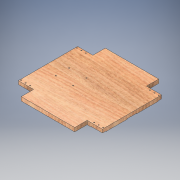
# Autodesk Inventor part: BottomPlateV1
Saved by Autodesk Inventor 2017 (Build 210142000, 142)
## iProperties
Created: 2017-01-25
Part Number: BottomPlateV1
Material: Wood (Birch)
Document SubType Name: Modeling
Designer: Naga
Density: 0.55 g/cm^3
Appearance: Birch - Natural Polished
Author: Naga
Autodesk Inventor part; units mm, degrees
ref_plane "YZ Plane" through (0, 0, 0) normal (1, 0, 0) x (0, 1, 0)
ref_plane "XZ Plane" through (0, 0, 0) normal (0, 1, 0) x (-1, 0, 0)
ref_plane "XY Plane" through (0, 0, 0) normal (0, 0, 1) x (1, 0, 0)
sketch "Sketch1" plane through (0, 0, 0) normal (0, 1, 0) x (-1, 0, 0)
  line L0 (-279.4, -127.4986) -> (-279.4, -151.8986)
  line L1 (-277.4, -125.4986) -> (-174.3, -125.4986)
  line L2 (-174.3, -153.8986) -> (-277.4, -153.8986)
  circle A0 centre (-275.8, -47.0543) radius 1.25
  circle A1 centre (-261, -47.0543) radius 1.25
  circle A2 centre (-246.2, -47.0543) radius 1.25
  circle A3 centre (-261, -232.44) radius 1.25
  circle A4 centre (-18.4, -47.0543) radius 1.25
  circle A5 centre (-48.23, -117.9957) radius 1.778
  circle A6 centre (-48.23, -162.1917) radius 1.778
  circle A7 centre (-105.38, -162.1917) radius 1.778
  circle A8 centre (-105.38, -117.9957) radius 1.778
  line L3 (0, 0) -> (-279.4, 0)
  line L4 (-279.4, 0) -> (-279.4, -279.4)
  line L5 (-279.4, -279.4) -> (0, -279.4)
  line L6 (0, -279.4) -> (0, 0)
  line L7 (-279.4, 0) -> (-228.6, 0)
  line L8 (-228.6, 0) -> (-228.6, -41.275)
  line L9 (-228.6, -41.275) -> (-279.4, -41.275)
  line L10 (-279.4, -41.275) -> (-279.4, 0)
  line L11 (-279.4, -279.4) -> (-228.6, -279.4)
  line L12 (-228.6, -279.4) -> (-228.6, -238.125)
  line L13 (-228.6, -238.125) -> (-279.4, -238.125)
  line L14 (-279.4, -238.125) -> (-279.4, -279.4)
  line L15 (0, -279.4) -> (-50.8, -279.4)
  line L16 (-50.8, -279.4) -> (-50.8, -238.125)
  line L17 (-50.8, -238.125) -> (0, -238.125)
  line L18 (0, -238.125) -> (0, -279.4)
  line L19 (0, 0) -> (-50.8, 0)
  line L20 (-50.8, 0) -> (-50.8, -41.275)
  line L21 (-50.8, -41.275) -> (0, -41.275)
  line L22 (0, -41.275) -> (0, 0)
  arc A9 (-174.3, -153.6986) -> (-174.3, -125.6986) centre (-182.3, -139.6986) ccw
  line L23 (-162.35, -123.8236) -> (-289.35, -123.8236)
  line L24 (-289.35, -123.8236) -> (-289.35, -155.5736)
  line L25 (-289.35, -155.5736) -> (-162.35, -155.5736)
  line L26 (-162.35, -155.5736) -> (-162.35, -123.8236)
  line L27 (-162.35, -123.8236) -> (-289.35, -155.5736) construction
  line L28 (-289.35, -123.8236) -> (-162.35, -155.5736) construction
  line L29 (-280.05, -238.79) -> (-241.95, -238.79)
  line L30 (-241.95, -238.79) -> (-241.95, -226.09)
  line L31 (-241.95, -226.09) -> (-280.05, -226.09)
  line L32 (-280.05, -226.09) -> (-280.05, -238.79)
  line L33 (-280.05, -238.79) -> (-241.95, -226.09) construction
  line L34 (-241.95, -238.79) -> (-280.05, -226.09) construction
  circle A10 centre (-261, -232.44) radius 1.5875
  circle A11 centre (-246.2, -232.44) radius 1.5875
  circle A12 centre (-275.8, -232.44) radius 1.5875
  line L35 (-261, -47.0543) -> (-261, -232.44)
  line L36 (-261, -232.44) -> (-18.4, -232.44)
  circle A13 centre (-261, -47.0454) radius 1.5875
  line L37 (-280.05, -53.3954) -> (-241.95, -53.3954)
  line L38 (-241.95, -53.3954) -> (-241.95, -40.6954)
  line L39 (-241.95, -40.6954) -> (-280.05, -40.6954)
  circle A14 centre (-246.2, -47.0454) radius 1.5875
  line L40 (-280.05, -40.6954) -> (-280.05, -53.3954)
  circle A15 centre (-275.8, -47.0454) radius 1.5875
  circle A16 centre (-18.4046, -232.44) radius 1.5875
  line L41 (-37.4546, -238.79) -> (0.6454, -238.79)
  line L42 (0.6454, -238.79) -> (0.6454, -226.09)
  line L43 (0.6454, -226.09) -> (-37.4546, -226.09)
  circle A17 centre (-3.6046, -232.44) radius 1.5875
  line L44 (-37.4546, -226.09) -> (-37.4546, -238.79)
  circle A18 centre (-33.2046, -232.44) radius 1.5875
  circle A19 centre (-18.4046, -47.0454) radius 1.5875
  line L45 (-37.4546, -53.3954) -> (0.6454, -53.3954)
  line L46 (0.6454, -53.3954) -> (0.6454, -40.6954)
  line L47 (0.6454, -40.6954) -> (-37.4546, -40.6954)
  circle A20 centre (-3.6046, -47.0454) radius 1.5875
  line L48 (-37.4546, -40.6954) -> (-37.4546, -53.3954)
  circle A21 centre (-33.2046, -47.0454) radius 1.5875
  point P0 (-225.85, -139.6986)
  dimension "d4" = 279.4
  dimension "d5" = 279.4
  dimension "d6" = 50.8
  dimension "d7" = 41.275
  dimension "d8" = 50.8
  dimension "d9" = 41.275
  dimension "d10" = 50.8
  dimension "d11" = 41.275
  dimension "d12" = 41.275
  dimension "d13" = 127
  dimension "d14" = 31.75
  dimension "d15" = 38.1
  dimension "d16" = 12.7
  dimension "d17" = 3.175
  dimension "d18" = 185.3946
  dimension "d19" = 242.5954
  constraints: 98 end point, 22 centre point, 14 parallel, 9 perpendicular, 8 horizontal, 4 midpoint, 2 point on circle, 1 coincident, 1 point on line, 1 vertical, 42 other
  measures "d4" distance of L5.end L4.end
  measures "d5" distance of L4.end L3.end
  measures "d6" distance of L8.end L9.end
  measures "d7" distance of L7.end L8.end
  measures "d8" distance of L13.end L12.end
  measures "d9" distance of L12.end L11.end
  measures "d10" distance of L16.end L17.end
  measures "d11" distance of L15.end L16.end
  measures "d12" distance of L20.end L19.end
  measures "d13" distance of L25.end L24.end
  measures "d14" distance of L24.end L23.end
  measures "d15" distance of L31.end L30.end
  measures "d16" distance of L30.end L29.end
  measures "d17" diameter of A10
  measures "d18" distance of L35.end A13.centre
  measures "d19" distance of L35.end A16.centre
extrude "Extrusion1" add sketch "Sketch1" along normal blind 12.7 contours L4 L23 L35 L25 L0 | L4 L37 L35 L23 | L25 L35 L31 L4 | L4 L9 L38 L37 | L35 L37 L38 L9 L8 L3 L20 L21 L48 L45 L6 L43 L44 L36 L30 L31 L25 L26 L23 | L23 L26 L25 L35 | L31 L35 A10 L36 A11 L30 L13 L4 | L31 L30 L36 A11 A10 L35 | L30 L36 L44 L17 L16 L5 L12 L13 | L44 L43 L6 L17 | L21 L6 L45 L48
sketch "Sketch3" plane through (0, 0, 0) normal (0, 1, 0) x (-1, 0, 0)
  line L0 (-279.4, -127.4986) -> (-279.4, -151.8986)
  line L1 (-277.4, -125.4986) -> (-174.3, -125.4986)
  line L2 (-174.3, -153.8986) -> (-277.4, -153.8986)
  circle A0 centre (-246.2, -47.0543) radius 1.25
  circle A1 centre (-261, -232.44) radius 1.25
  circle A2 centre (-18.4, -47.0543) radius 1.25
  circle A3 centre (-48.23, -117.9957) radius 1.778
  circle A4 centre (-48.23, -162.1917) radius 1.778
  circle A5 centre (-105.38, -162.1917) radius 1.778
  circle A6 centre (-105.38, -117.9957) radius 1.778
  line L3 (0, 0) -> (-279.4, 0)
  line L4 (-279.4, 0) -> (-279.4, -279.4)
  line L5 (-279.4, -279.4) -> (0, -279.4)
  line L6 (0, -279.4) -> (0, 0)
  line L7 (-279.4, 0) -> (-228.6, 0)
  line L8 (-279.4, -41.275) -> (-279.4, 0)
  line L9 (-279.4, -279.4) -> (-228.6, -279.4)
  line L10 (-228.6, -279.4) -> (-228.6, -238.125)
  line L11 (-228.6, -238.125) -> (-279.4, -238.125)
  line L12 (-279.4, -238.125) -> (-279.4, -279.4)
  line L13 (0, -279.4) -> (-50.8, -279.4)
  line L14 (-50.8, -279.4) -> (-50.8, -238.125)
  line L15 (-50.8, -238.125) -> (0, -238.125)
  line L16 (0, -238.125) -> (0, -279.4)
  line L17 (0, 0) -> (-50.8, 0)
  line L18 (-50.8, 0) -> (-50.8, -41.275)
  line L19 (-50.8, -41.275) -> (0, -41.275)
  line L20 (0, -41.275) -> (0, 0)
  arc A7 (-174.3, -153.6986) -> (-174.3, -125.6986) centre (-182.3, -139.6986) ccw
  line L21 (-162.35, -123.8236) -> (-289.35, -123.8236)
  line L22 (-289.35, -123.8236) -> (-289.35, -155.5736)
  line L23 (-289.35, -155.5736) -> (-162.35, -155.5736)
  line L24 (-162.35, -155.5736) -> (-162.35, -123.8236)
  line L25 (-162.35, -123.8236) -> (-289.35, -155.5736) construction
  line L26 (-289.35, -123.8236) -> (-162.35, -155.5736) construction
  line L27 (-280.05, -238.79) -> (-241.95, -238.79)
  line L28 (-241.95, -238.79) -> (-241.95, -226.09)
  line L29 (-241.95, -226.09) -> (-280.05, -226.09)
  line L30 (-280.05, -226.09) -> (-280.05, -238.79)
  line L31 (-280.05, -238.79) -> (-241.95, -226.09) construction
  line L32 (-241.95, -238.79) -> (-280.05, -226.09) construction
  circle A8 centre (-261, -232.44) radius 1.5875
  circle A9 centre (-246.2, -232.44) radius 1.5875
  circle A10 centre (-275.8, -232.44) radius 1.5875
  line L33 (-261, -47.0543) -> (-261, -232.44)
  line L34 (-261, -232.44) -> (-18.4, -232.44)
  circle A11 centre (-261, -47.0454) radius 1.5875
  line L35 (-280.05, -53.3954) -> (-241.95, -53.3954)
  line L36 (-241.95, -53.3954) -> (-241.95, -40.6954)
  line L37 (-241.95, -40.6954) -> (-280.05, -40.6954)
  circle A12 centre (-246.2, -47.0454) radius 1.5875
  line L38 (-280.05, -40.6954) -> (-280.05, -53.3954)
  circle A13 centre (-275.8, -47.0454) radius 1.5875
  circle A14 centre (-18.4046, -232.44) radius 1.5875
  line L39 (-37.4546, -238.79) -> (0.6454, -238.79)
  line L40 (0.6454, -238.79) -> (0.6454, -226.09)
  line L41 (0.6454, -226.09) -> (-37.4546, -226.09)
  circle A15 centre (-3.6046, -232.44) radius 1.5875
  line L42 (-37.4546, -226.09) -> (-37.4546, -238.79)
  circle A16 centre (-33.2046, -232.44) radius 1.5875
  circle A17 centre (-18.4046, -47.0454) radius 1.5875
  line L43 (-37.4546, -53.3954) -> (0.6454, -53.3954)
  line L44 (0.6454, -53.3954) -> (0.6454, -40.6954)
  line L45 (0.6454, -40.6954) -> (-37.4546, -40.6954)
  circle A18 centre (-3.6046, -47.0454) radius 1.5875
  line L46 (-37.4546, -40.6954) -> (-37.4546, -53.3954)
  circle A19 centre (-33.2046, -47.0454) radius 1.5875
  point P0 (-225.85, -139.6986)
  dimension "d26" = 279.4
  dimension "d27" = 279.4
  dimension "d30" = 50.8
  dimension "d31" = 41.275
  dimension "d32" = 50.8
  dimension "d33" = 41.275
  dimension "d34" = 41.275
  dimension "d35" = 127
  dimension "d36" = 31.75
  dimension "d37" = 38.1
  dimension "d38" = 12.7
  dimension "d39" = 3.175
  dimension "d40" = 185.3946
  dimension "d41" = 242.5954
  constraints: 94 end point, 20 centre point, 12 parallel, 8 horizontal, 8 perpendicular, 4 midpoint, 2 point on circle, 1 coincident, 1 point on line, 1 vertical, 42 other
  measures "d26" distance of L5.end L4.end
  measures "d27" distance of L4.end L3.end
  measures "d30" distance of L11.end L10.end
  measures "d31" distance of L10.end L9.end
  measures "d32" distance of L14.end L15.end
  measures "d33" distance of L13.end L14.end
  measures "d34" distance of L18.end L17.end
  measures "d35" distance of L23.end L22.end
  measures "d36" distance of L22.end L21.end
  measures "d37" distance of L29.end L28.end
  measures "d38" distance of L28.end L27.end
  measures "d39" diameter of A8
  measures "d40" distance of L33.end A11.centre
  measures "d41" distance of L33.end A14.centre
extrude "Extrusion2" cut sketch "Sketch3" along normal blind 1.5875 contours L4 L21 L33 L23 L0 | L0 L4 L23 L22 L21 | L35 L38 L37 L4 | L4 L37 L36 L35 | L21 L24 L23 L33 | L29 L33 A8 L34 A9 L28 L11 L4 | L4 L27 L30 L29 | L11 L28 L27 L4 | L29 L28 L34 A9 A8 L33 | L42 L41 L6 L15 | L15 L6 L39 L42 | L41 L40 L39 L6 | L45 L44 L43 L6 | L6 L19 L46 L45 | L19 L6 L43 L46
body "Solid1"
